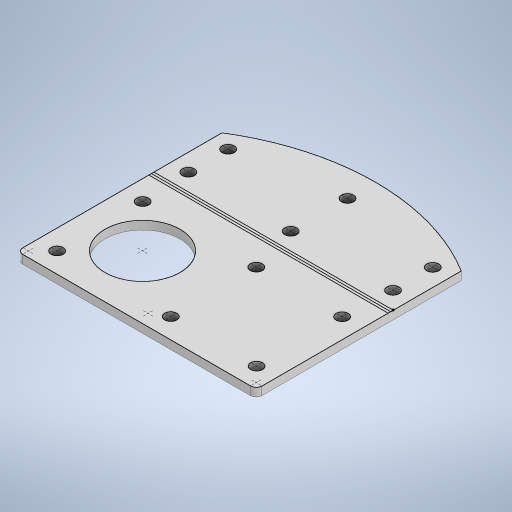
# Autodesk Inventor part: axis_2_bottom_L_frame(bottom)
Saved by Autodesk Inventor 2024.2 (Build 282272000, 272)
## iProperties
Created: 2024-01-11
Part Number: axis_2_bottom_L_frame(bottom)
Material: Generic
Document SubType Name: Modeling
Designer: chanh
Density: 1 g/cm^3
Appearance: Default
Author: chanh
Autodesk Inventor part; units mm, degrees
ref_plane "YZ Plane" through (0, 0, 0) normal (1, 0, 0) x (0, 1, 0)
ref_plane "XZ Plane" through (0, 0, 0) normal (0, 1, 0) x (-1, 0, 0)
ref_plane "XY Plane" through (0, 0, 0) normal (0, 0, 1) x (1, 0, 0)
sketch "Sketch1" plane through (0, 0, 0) normal (0, 1, 0) x (-1, 0, 0)
  line L0 (42.1, -59.7289) -> (0, -59.7289)
  circle A0 centre (31.1, -47.1593) radius 6.6
  circle A1 centre (38.6, -39.6343) radius 1.05
  circle A2 centre (38.6, -54.6843) radius 1.05
  circle A3 centre (18.6, -54.6843) radius 1.05
  circle A4 centre (18.6, -39.6343) radius 1.05
  circle A5 centre (3.5, -39.6343) radius 1.05
  circle A6 centre (3.5, -54.6843) radius 1.05
  circle A7 centre (3.05, -70.1786) radius 1.05
  circle A8 centre (3.05, -63.1786) radius 1.05
  circle A9 centre (21.05, -63.1786) radius 1.05
  circle A10 centre (21.05, -73.1786) radius 1.05
  circle A11 centre (39.05, -70.1786) radius 1.05
  circle A12 centre (39.05, -63.1786) radius 1.05
  arc A13 (42.1, -37.0893) -> (41.1, -36.0893) centre (41.1, -37.0893) ccw
  line L1 (41.1, -36.0893) -> (1, -36.0893)
  arc A14 (1, -36.0893) -> (0, -37.0893) centre (1, -37.0893) ccw
  arc A15 (0, -72.1318) -> (42.1, -72.1318) centre (21.05, -38.1186) ccw
  line L2 (0, -37.0893) -> (0, -72.1318)
  line L3 (42.1, -72.1318) -> (42.1, -37.0893)
  line L4 (42.1, -59.2793) -> (0, -59.2793)
  line L5 (0, -60.1786) -> (42.1, -60.1786)
  constraints: 16 centre point, 12 end point, 6 point on circle, 6 point on line, 4 horizontal, 2 vertical, 45 other
extrude "Extrusion1" add sketch "Sketch1" against normal blind 1.5
body "Solid1"
